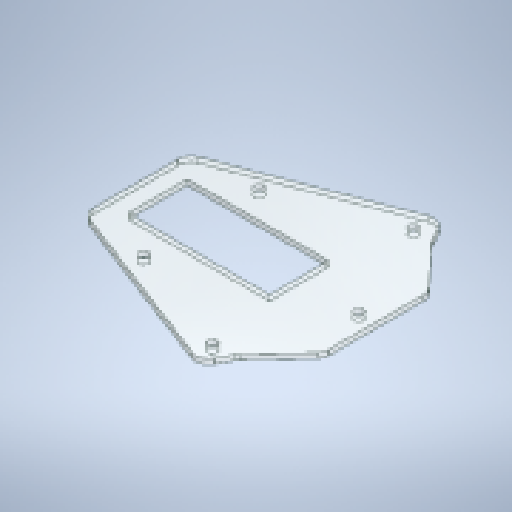
# Autodesk Inventor part: Screen Cover
Saved by Autodesk Inventor 2025 (Build 290162000, 162)
## iProperties
Created: 2025-04-19
Part Number: Screen Cover
Material: Generic
Document SubType Name: Modeling
Designer: User
Density: 1 g/cm^3
Appearance: Default
Author: User
Autodesk Inventor part; units mm, degrees
ref_plane "YZ Plane" through (0, 0, 0) normal (1, 0, 0) x (0, 1, 0)
ref_plane "XZ Plane" through (0, 0, 0) normal (0, 1, 0) x (-1, 0, 0)
ref_plane "XY Plane" through (0, 0, 0) normal (0, 0, 1) x (1, 0, 0)
sketch "Sketch1" plane through (0, 0, 0) normal (0, 1, 0) x (-1, 0, 0)
  line L0 (0, 0) -> (32.4, 0)
  line L1 (32.4, 0) -> (32.4, -13.5)
  line L2 (32.4, -13.5) -> (0, -13.5)
  line L3 (0, -13.5) -> (0, 0)
  line L4 (-5, 5) -> (37.4, 5)
  line L5 (37.4, 5) -> (37.4, -18.5)
  line L6 (37.4, -18.5) -> (-5, -18.5)
  line L7 (-5, -18.5) -> (-5, 5)
  line L8 (37.4, 5) -> (-5, 21.2758)
  line L9 (-5, 21.2758) -> (-5, -34.7758)
  line L10 (-5, -34.7758) -> (37.4, -18.5)
  line L11 (-5, 21.2758) -> (-8.0516, 15.5367)
  line L12 (-8.0516, 15.5367) -> (-17.644, 5.25)
  line L13 (-17.644, 5.25) -> (-17.644, -18.75)
  line L14 (-17.644, -18.75) -> (-8.0516, -29.0367)
  line L15 (-8.0516, -29.0367) -> (-5, -34.7758)
  point P0 (-5, -6.75)
  dimension "d0" = 32.4
  dimension "d1" = 13.5
  dimension "d2" = 5
  dimension "d5" = 21
  dimension "d6" = 21
  dimension "d8" = 28
  dimension "d9" = 28
  dimension "d11" = 6.5
  dimension "d12" = 24
  dimension "d13" = 6.5
  dimension "d15" = 165
  dimension "d16" = 165
  constraints: 32 end point, 4 parallel, 2 perpendicular, 2 vertical, 1 collinear, 1 horizontal, 1 midpoint, 3 other
  measures "d0" distance of L1.end L2.end
  measures "d1" distance of L0.end L1.end
  measures "d2" distance between parallel lines of L3 L7
  measures "d5" angle of L4 L8
  measures "d6" angle of L6 L10
  measures "d8" angle of L9 L11
  measures "d9" angle of L9 L15
  measures "d11" distance of L8.end L11.end
  measures "d12" distance of L12.end L13.end
  measures "d13" distance of L14.end L9.end
  measures "d15" angle of L11 L12
  measures "d16" angle of L15 L14
extrude "Extrusion1" add sketch "Sketch1" along normal blind 1.2
fillet "Fillet1" radius 3 8 edges at (5, 0.6, 21.2758) (17.644, 0.6, 5.25) (17.644, 0.6, -18.75) (5, 0.6, -34.7758) (8.0516, 0.6, -29.0367) (8.0516, 0.6, 15.5367) (-37.4, 0.6, 5) (-37.4, 0.6, -18.5)
sketch "Sketch2" plane through (0, 1.2, 0) normal (0, 1, 0) x (1, 0, 0)
  circle A0 centre (3.1296, -16.2733) radius 1.1
  circle A1 centre (3.1296, 29.7733) radius 1.1
  circle A2 centre (13.644, 6.75) radius 1.1
  circle A3 centre (-22.4, -6.4734) radius 1.1
  circle A4 centre (-22.4, 19.9734) radius 1.1
  arc A5 (-35.4751, 19.2389) -> (-37.4, 16.4382) centre (-34.4, 16.4382) ccw projected
  line L0 (-37.4, 16.4382) -> (-37.4, -2.9382) projected
  arc A6 (-37.4, -2.9382) -> (-35.4751, -5.7389) centre (-34.4, -2.9382) ccw projected
  line L1 (-35.4751, -5.7389) -> (2.5221, -20.3247) projected
  arc A7 (2.5221, -20.3247) -> (6.2461, -18.9323) centre (3.5972, -17.5239) ccw projected
  line L2 (6.2461, -18.9323) -> (7.8661, -15.8854) projected
  arc A8 (8.3209, -15.2478) -> (7.8661, -15.8854) centre (10.515, -17.2938) ccw projected
  line L3 (8.3209, -15.2478) -> (16.8381, -6.1143) projected
  arc A9 (16.8381, -6.1143) -> (17.644, -4.0683) centre (14.644, -4.0683) ccw projected
  line L4 (17.644, -4.0683) -> (17.644, 17.5683) projected
  arc A10 (17.644, 17.5683) -> (16.8381, 19.6143) centre (14.644, 17.5683) ccw projected
  line L5 (16.8381, 19.6143) -> (8.3209, 28.7478) projected
  arc A11 (7.8661, 29.3854) -> (8.3209, 28.7478) centre (10.515, 30.7938) ccw projected
  line L6 (7.8661, 29.3854) -> (6.2461, 32.4323) projected
  arc A12 (6.2461, 32.4323) -> (2.5221, 33.8247) centre (3.5972, 31.0239) ccw projected
  line L7 (2.5221, 33.8247) -> (-35.4751, 19.2389) projected
  line L8 (0, 0) -> (-32.4, 0) projected
  line L9 (-32.4, 0) -> (-32.4, 13.5) projected
  line L10 (-32.4, 13.5) -> (0, 13.5) projected
  line L11 (0, 13.5) -> (0, 0) projected
  point P0 (17.644, 6.75)
  dimension "d18" = 2.2
  dimension "d19" = 2.2
  dimension "d20" = 2.2
  dimension "d21" = 2.2
  dimension "d22" = 2.2
  dimension "d23" = 4
  dimension "d25" = 15
  dimension "d26" = 4
  dimension "d27" = 4
  dimension "d28" = 4
  dimension "d29" = 4
  dimension "d30" = 4
  constraints: 5 centre point, 2 vertical alignment, 1 horizontal alignment, 1 midpoint
  measures "d18" diameter of A0
  measures "d19" diameter of A1
  measures "d20" diameter of A2
  measures "d21" diameter of A3
  measures "d22" diameter of A4
  measures "d23" distance from line of A2.centre L4
  measures "d25" distance from line of A3.centre L0
  measures "d26" distance from line of A3.centre L1
  measures "d27" distance from line of A0.centre L2
  measures "d28" distance from line of A0.centre L1
  measures "d29" distance from line of L7 A1.centre
  measures "d30" distance from line of L7 A4.centre
extrude "Extrusion2" cut sketch "Sketch2" against normal up to surface (1.2 mm away) contours A0 | A1 | A2 | A3 | A4
equation "\"d6\" = d5"
equation "\"d9\" = d8"
equation "\"d13\" = d11"
equation "\"d16\" = d15"
equation "\"d23\" = d28"
equation "\"d26\" = d28"
equation "\"d27\" = d28"
equation "\"d29\" = d28"
equation "\"d30\" = d26"
equation "\"d31\" = d20"
body "Solid1"
